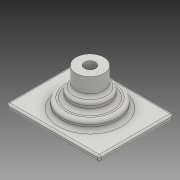
# Autodesk Inventor part: antena_up
Saved by Autodesk Inventor 2018 (Build 220112000, 112)
## iProperties
Created: 2018-11-22
Part Number: antena_up
Material: Genérico
Document SubType Name: Modeling
Designer: becar
Density: 1 g/cm^3
Appearance: Valor por defecto
Author: becar
Autodesk Inventor part; units mm, degrees
ref_plane "YZ Plane" through (0, 0, 0) normal (1, 0, 0) x (0, 1, 0)
ref_plane "XZ Plane" through (0, 0, 0) normal (0, 1, 0) x (-1, 0, 0)
ref_plane "XY Plane" through (0, 0, 0) normal (0, 0, 1) x (1, 0, 0)
sketch "Boceto1" plane through (0, 0, 0) normal (0, 0, 1) x (1, 0, 0)
  line L0 (0, 0) -> (0, 40)
  line L1 (0, 40) -> (50, 40)
  line L2 (50, 40) -> (50, 0)
  line L3 (50, 0) -> (0, 0)
  dimension "d0" = 40
  dimension "d1" = 50
  constraints: 8 end point, 3 perpendicular, 1 vertical
  measures "d0" distance of L0.start L0.end
  measures "d1" distance of L0.end L1.end
extrude "Extrusión1" add sketch "Boceto1" along normal blind 3
sketch "Boceto2" plane through (0, 0, 3) normal (0, 0, 1) x (1, 0, 0)
  line L0 (50, 40) -> (0, 40) projected
  line L1 (0, 0) -> (50, 0) projected
  circle A0 centre (25, 20) radius 15
  dimension "d4" = 30
  constraints: 1 centre point
  measures "d4" diameter of A0
extrude "Extrusión2" add sketch "Boceto2" along normal blind 5
sketch "Boceto3" plane through (25, 20, 8) normal (0, 0, 1) x (1, 0, 0)
  circle A0 centre (0, 0) radius 3
  circle A1 centre (0, 0) radius 7.5
  point P0 (-25, -20)
  dimension "d8" = 6
  dimension "d9" = 15
  constraints: 2 centre point, 1 coincident
  measures "d8" diameter of A0
  measures "d9" diameter of A1
extrude "Extrusión3" add sketch "Boceto3" along normal blind 15
sketch "Boceto4" plane through (25, 20, 8) normal (0, 0, 1) x (1, 0, 0)
  circle A0 centre (0, 0) radius 10
  point P0 (-25, -20)
  dimension "d12" = 20
  constraints: 1 centre point
  measures "d12" diameter of A0
extrude "Extrusión4" add sketch "Boceto4" along normal blind 5
fillet "Empalme1" radius 2 5 edges at (17.5, 20, 13) (15, 20, 13) (15, 20, 8) (10, 20, 8) (10, 20, 3)
fillet "Empalme2" radius 1 12 edges at (25, 0, 3) (50, 20, 3) (25, 0, 0) (50, 20, 0) (50, 0, 1.5) (0, 20, 3) (0, 20, 0) (0, 40, 1.5) (25, 40, 0) (25, 40, 3) (0, 0, 1.5) (50, 40, 1.5)
sketch "Boceto5" plane through (25, 20, 23) normal (0, 0, 1) x (1, 0, 0)
  circle A0 centre (0, 0) radius 3
  point P0 (-25, -20)
  constraints: 1 centre point
extrude "Extrusión5" cut sketch "Boceto5" against normal blind 20
